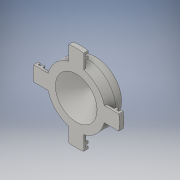
# Autodesk Inventor part: TopV2
Saved by Autodesk Inventor 2016 (Build 200138000, 138)
## iProperties
Created: 2016-01-09
Part Number: TopV2
Material: Generic
Document SubType Name: Modeling
Designer: bryan
Density: 1 g/cm^3
Appearance: Default
Author: bryan
Autodesk Inventor part; units mm, degrees
ref_plane "YZ Plane" through (0, 0, 0) normal (1, 0, 0) x (0, 1, 0)
ref_plane "XZ Plane" through (0, 0, 0) normal (0, 1, 0) x (-1, 0, 0)
ref_plane "XY Plane" through (0, 0, 0) normal (0, 0, 1) x (1, 0, 0)
sketch "Sketch1" plane through (0, 0, 0) normal (0, 1, 0) x (-1, 0, 0)
  point P0 (0, 0)
sketch "Sketch2" plane through (0, 0, 0) normal (0, 1, 0) x (-1, 0, 0)
  point P0 (0, 0)
sketch "Sketch3" plane through (0, 0, 0) normal (1, 0, 0) x (0, 1, 0)
  line L0 (0, 0) -> (635, 0) construction
  line L1 (0, 0) -> (0, 76.2) construction
  line L2 (0, 76.2) -> (635, 76.2) construction
  arc A0 (635, 0) -> (999.7931, 181.5955) centre (635, 457.2) ccw construction
  arc A1 (635, 76.2) -> (938.9942, 227.5296) centre (635, 457.2) ccw construction
  arc A2 (938.9942, 227.5296) -> (1066.8, 584.2) centre (432.3372, 610.3136) ccw construction
  arc A3 (999.7931, 181.5955) -> (1136.1393, 508) centre (432.3372, 610.3136) ccw construction
  line L3 (1397, 584.2) -> (1397, 508) construction
  line L4 (1397, 508) -> (1136.1393, 508) construction
  line L5 (1066.8, 584.2) -> (1320.8, 584.2) construction
  line L6 (1320.8, 584.2) -> (1320.8, 685.8) construction
  line L7 (1320.8, 685.8) -> (1397, 685.8) construction
  line L8 (1397, 685.8) -> (1397, 584.2) construction
  line L9 (635, 0) -> (1103.7061, 0) construction
  line L10 (1103.7061, 0) -> (1397, 508) construction
  line L11 (0, 152.4) -> (635, 152.4)
  arc A4 (635, 152.4) -> (878.1954, 273.4637) centre (635, 457.2) ccw
  arc A5 (878.1954, 273.4637) -> (990.5267, 584.2) centre (432.3372, 610.3136) ccw
  line L12 (990.5267, 584.2) -> (990.5267, 939.8)
  line L13 (990.5267, 939.8) -> (914.3267, 939.8)
  line L14 (914.3267, 939.8) -> (914.3267, 586.0467) construction
  line L15 (635, 228.6) -> (0, 228.6) construction
  line L16 (0, 228.6) -> (0, 152.4)
  arc A6 (817.3965, 319.3977) -> (914.3267, 586.0467) centre (432.3372, 610.3136) ccw
  arc A7 (635, 228.6) -> (817.3965, 319.3977) centre (635, 457.2) ccw construction
  line L17 (914.3267, 939.8) -> (711.2, 939.8)
  line L18 (711.2, 939.8) -> (0, 228.6)
  dimension "d0" = 1397
  dimension "d1" = 76.2
  dimension "d3" = 635
  dimension "d4" = 101.6
  dimension "d5" = 76.2
  dimension "d6" = 254
  dimension "d7" = 685.8
  dimension "d8" = 60
  dimension "d9" = 635
  dimension "d10" = 381
  dimension "d32" = 76.2
  dimension "d33" = 355.6
  dimension "d34" = 45
  constraints: 38 end point, 16 point on circle, 8 centre point, 8 tangent, 7 perpendicular, 6 concentric, 6 horizontal, 4 equal length, 2 point on line, 2 vertical, 1 parallel
  measures "d0" distance between parallel lines of L1 L3
  measures "d1" distance of L0.start L1.end
  measures "d3" distance of L1.end L2.end
  measures "d4" distance of L5.end L6.end
  measures "d5" distance between parallel lines of L5 L4
  measures "d6" distance of L5.start L5.end
  measures "d7" distance between parallel lines of L7 L0
  measures "d8" angle of L10 L9
  measures "d9" radius of A2
  measures "d10" radius of A1
  measures "d32" distance between parallel lines of L11 L2
  measures "d33" distance between parallel lines of L13 L5
  measures "d34" angle of L18 L17
revolve "Revolution1" add sketch "Sketch3" angle 360 about axis through (0, 0, 0) along (0, 0, 1)
sketch "Sketch7" plane through (0, 0, 939.8) normal (0, 0, 1) x (1, 0, 0)
  circle A0 centre (0, 0) radius 990.5267
  circle A1 centre (0, 0) radius 1473.2
  circle A2 centre (0, 0) radius 990.5267 projected
  dimension "d35" = 2946.4
  constraints: 2 centre point, 2 coincident, 1 concentric
  measures "d35" diameter of A1
extrude "Extrusion4" add sketch "Sketch7" against normal blind 76.2
sketch "Sketch8" plane through (0, 0, 863.6) normal (0, 0, -1) x (-1, 0, 0)
  circle A0 centre (0, 0) radius 1473.2
  circle A1 centre (0, 0) radius 1398.27
  circle A2 centre (0, 0) radius 1319.53
  circle A3 centre (0, 0) radius 1243.33
  circle A4 centre (0, 0) radius 1473.2 projected
  dimension "d38" = 74.93
  dimension "d39" = 76.2
  dimension "d40" = 78.74
  constraints: 4 centre point, 4 coincident, 1 concentric
  measures "d38" radial gap between concentric circles of A0 A1
  measures "d39" radial gap between concentric circles of A3 A2
  measures "d40" radial gap between concentric circles of A2 A1
extrude "Extrusion5" add sketch "Sketch8" along normal blind 76.2
sketch "Sketch9" plane through (0, 0, 863.6) normal (0, 0, -1) x (-1, 0, 0)
  circle A0 centre (0, 0) radius 990.5267
  circle A1 centre (0, 0) radius 990.5267 projected
  circle A2 centre (0, 0) radius 990.5267 projected
  line L0 (-957.4064, 254) -> (-1726.5763, 254)
  line L1 (-1726.5763, 254) -> (-1726.5763, 2407.0489)
  line L2 (-1726.5763, 2407.0489) -> (-254, 2407.0489)
  line L3 (-254, 2407.0489) -> (-254, 957.4064)
  line L4 (254, 957.4064) -> (254, 2407.0489)
  line L5 (254, 2407.0489) -> (1885.1535, 2407.0489)
  line L6 (1885.1535, 2407.0489) -> (1885.1535, 254)
  line L7 (1885.1535, 254) -> (957.4064, 254)
  line L8 (-957.4064, -254) -> (-1726.5763, -254)
  line L9 (-1726.5763, -254) -> (-1726.5763, -2420.2811)
  line L10 (-1726.5763, -2420.2811) -> (-254, -2420.2811)
  line L11 (-254, -2420.2811) -> (-254, -957.4064)
  line L12 (254, -957.4064) -> (254, -2461.2485)
  line L13 (254, -2461.2485) -> (1932.9488, -2461.2485)
  line L14 (1932.9488, -2461.2485) -> (1932.9488, -254)
  line L15 (1932.9488, -254) -> (957.4064, -254)
  point P0 (254, -1709.3275)
  dimension "d43" = 508
  dimension "d44" = 508
  dimension "d45" = 508
  dimension "d46" = 508
  dimension "d47" = 254
  dimension "d48" = 254
  constraints: 32 end point, 5 horizontal, 5 perpendicular, 5 point on circle, 5 vertical, 2 collinear, 2 point on line, 1 centre point, 1 coincident, 1 midpoint, 10 other
  measures "d43" distance between parallel lines of L4 L3
  measures "d44" distance between parallel lines of L12 L11
  measures "d45" distance between parallel lines of L15 L7
  measures "d46" distance between parallel lines of L8 L0
  measures "d47" distance from line of L0 point (0, 0)
  measures "d48" distance from line of point (0, 0) L4
extrude "Extrusion6" cut sketch "Sketch9" against normal blind 127 and the other way blind 127 contours A0 L4 L5 L6 L7 | L15 L14 L13 L12 A0 | A0 L0 L1 L2 L3 | L11 L10 L9 L8 A0
body "Solid1"
